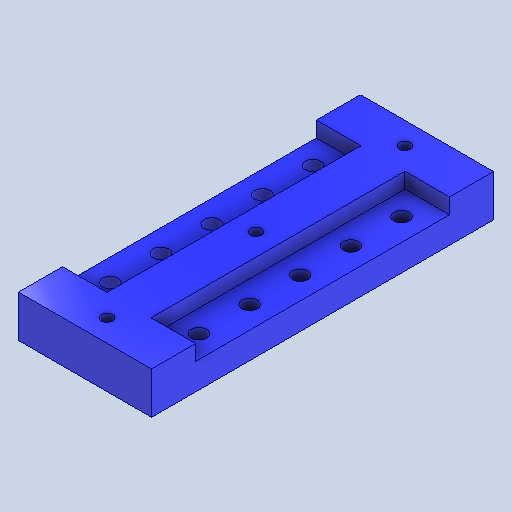
# Autodesk Inventor part: CO-1-1-CellSpacerMountMiddle
Saved by Autodesk Inventor 2023 (Build 270158000, 158)
## iProperties
Created: 2023-01-22
Part Number: CO-1-1-CellSpacerMountMiddle
Material: Generic
Document SubType Name: Modeling
Designer: asach
Density: 1 g/cm^3
Appearance: Blue - Wall Paint - Glossy
Author: asach
Autodesk Inventor part; units mm, degrees
ref_plane "YZ Plane" through (0, 0, 0) normal (1, 0, 0) x (0, 1, 0)
ref_plane "XZ Plane" through (0, 0, 0) normal (0, 1, 0) x (-1, 0, 0)
sketch "Sketch1" plane through (0, 0, 0) normal (0, 1, 0) x (-1, 0, 0)
  line L0 (0, 0) -> (40.2, 0)
  line L1 (40.2, 0) -> (40.2, -155.2)
  line L2 (40.2, -155.2) -> (0, -155.2)
  line L3 (0, -155.2) -> (0, 0)
  line L4 (0, -20) -> (20.2, -20)
  line L5 (20.2, -20) -> (20.2, -135.2)
  line L6 (20.2, -135.2) -> (0, -135.2)
  line L7 (0, -135.2) -> (0, -20)
  line L8 (10.1, -135.2) -> (10.1, -20) construction
  line L9 (20.2, -77.6) -> (0, -77.6) construction
  circle A0 centre (10.1, -77.6) radius 3.5
  line L10 (0, -54.6) -> (20.2, -54.6) construction
  line L11 (20.2, -31.6) -> (0, -31.6) construction
  circle A1 centre (10.1, -54.6) radius 3.5
  circle A2 centre (10.1, -31.6) radius 3.5
  circle A3 centre (10.1, -100.6) radius 3.5
  circle A4 centre (10.1, -123.6) radius 3.5
  line L12 (40.2, -155.2) -> (20.2, -135.2) construction
  line L13 (30.2, -155.2) -> (30.2, 0) construction
  line L14 (20.2, -20) -> (40.2, 0) construction
  circle A5 centre (30.2, -145.2) radius 2.6
  circle A6 centre (30.2, -10) radius 2.6
  circle A7 centre (30.2, -77.6) radius 2.6
  point P0 (0, -135.2)
  dimension "d0" = 115.2
  dimension "d1" = 20.2
  dimension "d2" = 7
  dimension "d3" = 23
  dimension "d4" = 23
  dimension "d11" = 20
  dimension "d12" = 20
  dimension "d13" = 20
  dimension "d14" = 5.2
  constraints: 30 end point, 10 midpoint, 8 centre point, 8 point on line, 5 perpendicular, 4 equal radius, 4 parallel, 2 horizontal, 2 symmetric about line, 2 other
  measures "d0" distance of L4.end L5.end
  measures "d1" distance of L5.end L6.end
  measures "d2" diameter of A0
  measures "d3" distance between parallel lines of L10 L9
  measures "d4" distance between parallel lines of L11 L10
  measures "d11" distance between parallel lines of L1 L5
  measures "d12" distance between parallel lines of L6 L2
  measures "d13" distance between parallel lines of L0 L4
  measures "d14" diameter of A5
extrude "Extrusion1" add sketch "Sketch1" along normal blind 12 contours L4 L5 L6 L3
extrude "Extrusion2" add sketch "Sketch1" along normal blind 2 contours A0 | A1 | A2 | A3 | A4
extrude "Extrusion3" add sketch "Sketch1" along normal blind 19 contours L0 L1 L2 L3 L6 L5 L4
sketch "Sketch2" plane through (0, 19, 0) normal (0, 1, 0) x (1, 0, 0)
  line L0 (-40.2, 155.2) -> (-40.2, 0) projected
  line L1 (-40.2, 0) -> (0, 0) projected
  line L2 (0, 0) -> (0, 20) projected
  line L3 (0, 20) -> (-20.2, 20) projected
  line L4 (-20.2, 20) -> (-20.2, 135.2) projected
  line L5 (-20.2, 135.2) -> (0, 135.2) projected
  line L6 (0, 135.2) -> (0, 155.2) projected
  line L7 (0, 155.2) -> (-40.2, 155.2) projected
  circle A0 centre (-30.2, 77.6) radius 2.6 projected
  circle A1 centre (-30.2, 145.2) radius 2.6 projected
  circle A2 centre (-30.2, 10) radius 2.6 projected
  line L8 (-30.2, 10) -> (-30.2, 145.2)
  constraints: 2 end point, 1 vertical
ref_plane "Work Plane1" through (-30.2, 19, -10) normal (1, 0, 0) x (0, 0, -1)
mirror "Mirror1" about plane through (-30.2, 19, -10) normal (1, 0, 0) of "Extrusion3", "Extrusion2", "Extrusion1"
equation "\"d1\" = screwTabWidth + tolerance"
equation "\"d2\" = insertDiameter"
equation "\"d11\" = screwTabWidth"
equation "\"d12\" = screwTabWidth"
equation "\"d13\" = screwTabWidth"
equation "\"d14\" = screwDiameter + tolerance"
equation "\"d5\" = insertPadding + insertLength"
equation "\"d7\" = insertPadding"
equation "\"d9\" = insertLength + insertPadding + baseThickness"
equation "\"insertDiameter\" = 7"
equation "\"insertLength\" = 10"
equation "\"insertPadding\" = 2"
equation "\"tolerance\" = 0.2"
equation "\"cellSpacing_1\" = 1"
equation "\"screwDiameter_1\" = 5"
equation "\"baseThickness_1\" = 7"
equation "\"tabThickness_1\" = 0.8"
equation "\"batteryBoxWidth\" = 162"
equation "\"sheetMetalThickness\" = 3.175"
equation "\"screwTabWidth\" = 20"
equation "\"screwDiameter\" = 5"
equation "\"baseThickness\" = 7"
body "Solid1"
